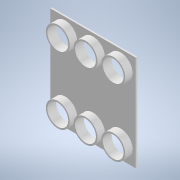
# Autodesk Inventor part: vial holder 2
Saved by Autodesk Inventor 2022 (Build 260153000, 153)
## iProperties
Created: 2022-05-06
Part Number: vial holder 2
Material: Generic
Document SubType Name: Modeling
Designer: efred
Density: 1 g/cm^3
Appearance: Default
Author: efred
Autodesk Inventor part; units mm, degrees
ref_plane "YZ Plane" through (0, 0, 0) normal (1, 0, 0) x (0, 1, 0)
ref_plane "XZ Plane" through (0, 0, 0) normal (0, 1, 0) x (-1, 0, 0)
ref_plane "XY Plane" through (0, 0, 0) normal (0, 0, 1) x (1, 0, 0)
sketch "Sketch1" plane through (0, 0, 0) normal (0, 0, 1) x (1, 0, 0)
  circle A0 centre (41.875, 108.01) radius 13.75 construction
  circle A1 centre (4.875, 108.01) radius 13.75 construction
  circle A2 centre (-32.125, 108.01) radius 13.75 construction
  circle A3 centre (41.875, 20.01) radius 13.75 construction
  circle A4 centre (4.875, 20.01) radius 13.75 construction
  circle A5 centre (-32.125, 20.01) radius 13.75 construction
  line L0 (61.875, 0.01) -> (-52.125, 0.01)
  line L1 (-52.125, 0.01) -> (-52.125, 128.01)
  line L2 (-52.125, 128.01) -> (61.875, 128.01)
  line L3 (61.875, 128.01) -> (61.875, 0.01)
  circle A6 centre (41.875, 20.01) radius 14.05
  circle A7 centre (4.875, 20.01) radius 14.05
  circle A8 centre (-32.125, 20.01) radius 14.05
  circle A9 centre (41.875, 108.01) radius 14.05
  circle A10 centre (4.875, 108.01) radius 14.05
  circle A11 centre (-32.125, 108.01) radius 14.05
  point P0 (0, 0)
  dimension "d0" = 20
  dimension "d1" = 20
  dimension "d2" = 20
  dimension "d3" = 20
  dimension "d4" = 0.3
  dimension "d5" = 0.3
  dimension "d6" = 0.3
  dimension "d7" = 0.3
  dimension "d8" = 0.3
  dimension "d9" = 0.3
  constraints: 8 end point, 6 centre point, 2 parallel, 1 horizontal, 1 perpendicular
  measures "d0" distance from line of A3.centre L3
  measures "d1" distance from line of L0 A3.centre
  measures "d2" distance from line of A5.centre L1
  measures "d3" distance from line of A2.centre L2
  measures "d4" radial gap between concentric circles of A3 A6
  measures "d5" radial gap between concentric circles of A4 A7
  measures "d6" radial gap between concentric circles of A5 A8
  measures "d7" radial gap between concentric circles of A0 A9
  measures "d8" radial gap between concentric circles of A1 A10
  measures "d9" radial gap between concentric circles of A2 A11
extrude "Extrusion1" add sketch "Sketch1" along normal blind 2
sketch "Sketch2" plane through (0, 0, 2) normal (0, 0, 1) x (1, 0, 0)
  line L0 (61.875, 128.01) -> (-52.125, 128.01) projected
  line L1 (-52.125, 128.01) -> (-52.125, 0.01) projected
  line L2 (-52.125, 0.01) -> (61.875, 0.01) projected
  line L3 (61.875, 0.01) -> (61.875, 128.01) projected
  circle A0 centre (-32.125, 108.01) radius 14.05 projected
  circle A1 centre (4.875, 108.01) radius 14.05 projected
  circle A2 centre (41.875, 108.01) radius 14.05 projected
  circle A3 centre (-32.125, 20.01) radius 14.05 projected
  circle A4 centre (4.875, 20.01) radius 14.05 projected
  circle A5 centre (41.875, 20.01) radius 14.05 projected
  circle A6 centre (41.875, 20.01) radius 16.05
  circle A7 centre (4.875, 20.01) radius 16.05
  circle A8 centre (-32.125, 20.01) radius 16.05
  circle A9 centre (41.875, 108.01) radius 16.05
  circle A10 centre (4.875, 108.01) radius 16.05
  circle A11 centre (-32.125, 108.01) radius 16.05
  point P0 (0, 0)
  dimension "d12" = 2
  dimension "d13" = 2
  dimension "d14" = 2
  dimension "d15" = 2
  dimension "d16" = 2
  dimension "d17" = 2
  constraints: 6 centre point
  measures "d12" radial gap between concentric circles of A5 A6
  measures "d13" radial gap between concentric circles of A4 A7
  measures "d14" radial gap between concentric circles of A3 A8
  measures "d15" radial gap between concentric circles of A2 A9
  measures "d16" radial gap between concentric circles of A1 A10
  measures "d17" radial gap between concentric circles of A0 A11
extrude "Extrusion2" add sketch "Sketch2" along normal blind 10 contours A6 | A7 | A8 | A9 | A10 | A11
equation "\"d5\" = d4"
equation "\"d6\" = d4"
equation "\"d7\" = d4"
equation "\"d8\" = d4"
equation "\"d9\" = d4"
body "Solid1"
